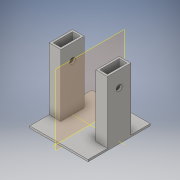
# Autodesk Inventor part: PostForLift
Saved by Autodesk Inventor 2016 SP1 (Build 200210100, 210)
## iProperties
Created: 2016-02-01
Part Number: PostForLift
Material: Generic
Document SubType Name: Modeling
Designer: steele
Density: 1 g/cm^3
Appearance: Default
Author: steele
Autodesk Inventor part; units mm, degrees
ref_plane "XZ Plane" through (0, 0, 0) normal (0, 1, 0) x (-1, 0, 0)
ref_plane "XY Plane" through (0, 0, 0) normal (0, 0, 1) x (1, 0, 0)
sketch "Sketch1" plane through (0, 0, 0) normal (0, 1, 0) x (-1, 0, 0)
  line L0 (47.625, 50.8) -> (-47.625, 50.8)
  line L1 (-47.625, 50.8) -> (-47.625, -50.8)
  line L2 (-47.625, -50.8) -> (47.625, -50.8)
  line L3 (47.625, -50.8) -> (47.625, 50.8)
  line L4 (47.625, 50.8) -> (-47.625, -50.8) construction
  line L5 (-47.625, 50.8) -> (47.625, -50.8) construction
  point P0 (0, 0)
  dimension "d0" = 95.25
  dimension "d1" = 101.6
  constraints: 12 end point, 2 midpoint, 2 parallel, 1 horizontal, 1 perpendicular
  measures "d0" distance of L0.start L0.end
  measures "d1" distance of L2.end L0.start
extrude "Extrusion1" add sketch "Sketch1" against normal blind 3.175
sketch "Sketch2" plane through (0, 0, 0) normal (0, 1, 0) x (1, 0, 0)
  line L0 (-47.625, -19.05) -> (-28.575, -19.05)
  line L1 (-28.575, -19.05) -> (-28.575, 19.05)
  line L2 (-28.575, 19.05) -> (-47.625, 19.05)
  line L3 (-47.625, 19.05) -> (-47.625, -19.05)
  line L4 (-47.625, -19.05) -> (-28.575, 19.05) construction
  line L5 (-28.575, -19.05) -> (-47.625, 19.05) construction
  line L6 (-44.45, -15.875) -> (-31.75, -15.875)
  line L7 (-31.75, -15.875) -> (-31.75, 15.875)
  line L8 (-31.75, 15.875) -> (-44.45, 15.875)
  line L9 (-44.45, 15.875) -> (-44.45, -15.875)
  line L10 (-44.45, -15.875) -> (-31.75, 15.875) construction
  line L11 (-31.75, -15.875) -> (-44.45, 15.875) construction
  line L12 (-47.625, 50.8) -> (47.625, 50.8) construction
  line L13 (0, 50.8) -> (0, -101.6) construction
  line L14 (47.625, -19.05) -> (28.575, -19.05)
  line L15 (28.575, -19.05) -> (28.575, 19.05)
  line L16 (28.575, 19.05) -> (47.625, 19.05)
  line L17 (47.625, 19.05) -> (47.625, -19.05)
  line L18 (44.45, -15.875) -> (31.75, -15.875)
  line L19 (31.75, -15.875) -> (31.75, 15.875)
  line L20 (31.75, 15.875) -> (44.45, 15.875)
  line L21 (44.45, 15.875) -> (44.45, -15.875)
  point P0 (0, 0)
  point P1 (-38.1, 0)
  dimension "d4" = 38.1
  dimension "d5" = 19.05
  dimension "d6" = 38.1
  dimension "d7" = 3.175
  dimension "d8" = 3.175
  constraints: 42 end point, 8 symmetric about line, 5 midpoint, 4 parallel, 2 horizontal, 2 perpendicular, 1 vertical
  measures "d4" distance of point (0, 0) point (-38.1, 0)
  measures "d5" distance of L0.start L0.end
  measures "d6" distance of L2.end L0.start
  measures "d7" distance between parallel lines of L0 L6
  measures "d8" distance between parallel lines of L9 L3
extrude "Extrusion2" add sketch "Sketch2" along normal blind 101.6
sketch "Sketch4" plane through (-47.625, -3.175, -50.8) normal (-1, 0, 0) x (0, 0, 1)
  line L0 (50.8, 3.175) -> (50.8, 93.283) construction
  circle A0 centre (50.8, 79.375) radius 4.7625
  line L1 (0, 3.175) -> (31.75, 3.175) projected
  dimension "d15" = 9.525
  dimension "d16" = 76.2
  constraints: 2 end point, 1 centre point, 1 point on line, 1 vertical
  measures "d15" diameter of A0
  measures "d16" distance from line of A0.centre L1
extrude "Extrusion4" cut sketch "Sketch4" against normal through all
equation "\"d0\" = BaseWidth"
equation "\"d1\" = BaseLength"
equation "\"d2\" = BaseThickness"
equation "\"d4\" = postCenterDistanceFromCenterOfBase"
equation "\"d5\" = postWidth"
equation "\"d6\" = postLength"
equation "\"d7\" = postThickness"
equation "\"d8\" = postThickness"
equation "\"d9\" = postHeight"
equation "\"d15\" = axelDiam"
equation "\"d16\" = axelHeightAbovePlate"
equation "\"BaseWidth\" = 95.25"
equation "\"BaseLength\" = 101.6"
equation "\"BaseThickness\" = 3.175"
equation "\"postWidth\" = 19.05"
equation "\"postLength\" = 38.1"
equation "\"postThickness\" = 3.175"
equation "\"postCenterDistanceFromCenterOfBase\" = 38.1"
equation "\"axelDiam\" = 9.525"
equation "\"axelHeightAbovePlate\" = 76.2"
equation "\"postHeight\" = 101.6"
body "Solid1"
